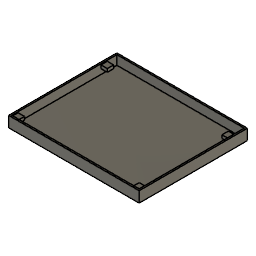
Carcasa Proyecto final V1 (Autodesk Fusion 360 design; units mm, degrees)
part number: 2026-09-21-08-55-22-859
Autodesk Fusion 360 part; units mm, degrees
sketch "Boceto1" plane through (0, 0, 0) normal (0, 0, 1) x (1, 0, 0)
  line L0 (0, 0) -> (-41, 0)
  line L1 (-41, 0) -> (-41, -34)
  line L2 (-41, -34) -> (0, -34)
  line L3 (0, -34) -> (0, 0)
  dimension "d1" = 34
  dimension "d2" = 41
  constraint horizontal L0
  constraint vertical L1
  constraint horizontal L2
  constraint vertical L3
  constraint coincident L0.start L3.end
  measures "d1" distance of L0.start L2.end
  measures "d2" distance of L0.start L0.end
extrude "Extruir1" add sketch "Boceto1" along normal blind 3.4 makes body 1
shell "Vaciado1" thickness 0.5 removed faces 1 at (-27.3333, -11.3333, 3.4) on bodies 1
sketch "Boceto2" plane through (0, 0, 0.5) normal (0, 0, 1) x (-1, 0, 0)
  line L0 (0.5, 33.5) -> (0.5, 0.5)
  line L1 (0.5, 0.5) -> (40.5, 0.5)
  line L2 (40.5, 0.5) -> (40.5, 33.5)
  line L3 (40.5, 33.5) -> (0.5, 33.5)
  line L4 (0.5, 0.5) -> (2.5, 0.5)
  line L5 (2.5, 0.5) -> (2.5, 2.5)
  line L6 (2.5, 2.5) -> (0.5, 2.5)
  line L7 (0.5, 2.5) -> (0.5, 0.5)
  dimension "d6" = 2
  dimension "d7" = 2
  constraint horizontal L4
  constraint vertical L5
  constraint horizontal L6
  constraint vertical L7
  constraint coincident L0.end L1.start
  measures "d6" distance of L0.end L4.end
  measures "d7" distance of L0.end L6.end
extrude "Extruir2" add sketch "Boceto2" along normal blind 1 contours L0 L1 L4 L5 L6 L7 bodies 1
delete_face "SuprimirCaras1" 3 faces at (-1.8333, -1.1667, 1.5) (-2.5, -1.1667, 0.8333) (-1.1667, -2.5, 1.1667) on bodies 1
sketch "Boceto3" plane through (0, 0, 0) normal (0, 0, 1) x (1, 0, 0)
  line L0 (2.5, 0) -> (4.5, 0)
  line L1 (4.5, 0) -> (4.5, -2)
  line L2 (4.5, -2) -> (2.5, -2)
  line L3 (2.5, -2) -> (2.5, 0)
  constraint horizontal L0
  constraint vertical L1
  constraint horizontal L2
  constraint vertical L3
extrude "Extruir3" add sketch "Boceto3" along normal blind 1 separate body makes body 2
move_body "Desplazar1" bodies 2 to x (1, 0, 0) y (0, 1, 0) z (0, 0, 1) at (-5, 0, 3)
move_body "Desplazar2" bodies 2 to x (1, 0, 0) y (0, 1, 0) z (0, 0, 1) at (0, -0.5, 0)
copy_body "CopiarPegarCuerpos1" bodies 2 makes body 3
copy_body "CopiarPegarCuerpos2" bodies 2 makes body 4
copy_body "CopiarPegarCuerpos3" bodies 2 makes body 5
move_body "Desplazar3" bodies 3 to x (1, 0, 0) y (0, 1, 0) z (0, 0, 1) at (-41, 0, 0)
move_body "Desplazar4" bodies 4 to x (1, 0, 0) y (0, 1, 0) z (0, 0, 1) at (0, -34, 0)
move_body "Desplazar5" bodies 5 to x (1, 0, 0) y (0, 1, 0) z (0, 0, 1) at (-41, -34, 0)
move_body "Desplazar6" bodies 3 to x (1, 0, 0) y (0, 1, 0) z (0, 0, 1) at (3, 0, 0)
move_body "Desplazar7" bodies 5 to x (1, 0, 0) y (0, 1, 0) z (0, 0, 1) at (3, 3, 0)
move_body "Desplazar8" bodies 4 to x (1, 0, 0) y (0, 1, 0) z (0, 0, 1) at (0, 3, 0)
move_body "Desplazar9" bodies 4 to x (1, 0, 0) y (0, 1, 0) z (0, 0, 1) at (0, 0, -1)
move_body "Desplazar10" bodies 4 to x (1, 0, 0) y (0, 1, 0) z (0, 0, 1) at (0, 0, 0.1)
move_body "Desplazar11" bodies 3 to x (1, 0, 0) y (0, 1, 0) z (0, 0, 1) at (0, 0, -0.9)
move_body "Desplazar12" bodies 5 to x (1, 0, 0) y (0, 1, 0) z (0, 0, 1) at (0, 0, -0.9)
move_body "Desplazar13" bodies 2 to x (1, 0, 0) y (0, 1, 0) z (0, 0, 1) at (0, 0, -0.9)
move_body "Desplazar14" bodies 3 to x (1, 0, 0) y (0, 1, 0) z (0, 0, 1) at (0, -3, 0)
move_body "Desplazar15" bodies 2 to x (1, 0, 0) y (0, 1, 0) z (0, 0, 1) at (0, -3, 0)
